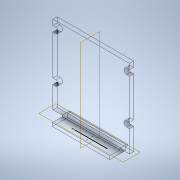
# Autodesk Inventor part: Xaar128
Saved by Autodesk Inventor 2022 (Build 260153000, 153)
## iProperties
Created: 2024-05-05
Part Number: Xaar128
Material: Generic
Document SubType Name: Modeling
Designer: raphael.hauk
Density: 1 g/cm^3
Appearance: Default
Author: raphael.hauk
Autodesk Inventor part; units mm, degrees
ref_plane "XY Plane" through (0, 0, 0) normal (0, 0, 1) x (1, 0, 0)
sketch "Sketch1" plane through (0, 0, 0) normal (0, 1, 0) x (-1, 0, 0)
  line L0 (0, -0.13) -> (17.417, -0.13)
  line L1 (17.417, -0.13) -> (17.417, 0.13)
  line L2 (17.417, 0.13) -> (0, 0.13)
  line L3 (0, 0.13) -> (0, -0.13)
  line L4 (-17.289, 0) -> (34.651, 0) construction
  line L5 (22.681, -3.5) -> (-5.169, -3.5)
  line L6 (-5.169, -3.5) -> (-5.169, 4)
  line L7 (-5.169, 4) -> (22.681, 4)
  line L8 (22.681, 4) -> (22.681, -3.5)
  line L9 (27.231, -2.85) -> (-9.869, -2.85) construction
  line L10 (-9.869, -2.85) -> (-9.869, -0.85) construction
  line L11 (-9.869, -0.85) -> (27.231, -0.85) construction
  line L12 (27.231, -0.85) -> (27.231, -2.85) construction
  point P0 (0, 0)
  dimension "d1" = 17.417
  dimension "d2" = 0.26
  dimension "d7" = 7.5
  dimension "d8" = 27.85
  dimension "d9" = 0.85
  dimension "d10" = 2
  dimension "d11" = 9.814
  dimension "d12" = 37.1
  dimension "d13" = 4.55
  dimension "d20" = 4.85
  constraints: 24 end point, 6 parallel, 3 horizontal, 3 perpendicular, 1 midpoint, 1 other
  measures "d1" distance of L0.start L0.end
  measures "d2" distance of L0.end L1.end
  measures "d7" distance of L7.end L5.start
  measures "d8" distance of L5.start L5.end
  measures "d9" distance between parallel lines of L11 L4
  measures "d10" distance of L9.end L10.end
  measures "d11" distance from line of L0.end L12
  measures "d12" distance of L9.start L9.end
  measures "d13" distance between parallel lines of L12 L8
  measures "d20" distance between parallel lines of L7 L11
ref_plane "Alu_Start_V" through (0, 2.27, 0) normal (0, 1, 0) x (-1, 0, 0)
sketch "Sketch2" plane through (0, 2.27, 0) normal (0, 1, 0) x (-1, 0, 0)
  line L0 (27.231, -2.85) -> (-9.869, -2.85) projected
  line L1 (27.231, -0.85) -> (27.231, -2.85) projected
  line L2 (-9.869, -0.85) -> (27.231, -0.85) projected
  line L3 (-9.869, -2.85) -> (-9.869, -0.85) projected
  point P0 (0, 0)
extrude "Extrusion2" add sketch "Sketch2" along normal blind 38
extrude "Extrusion3" add sketch "Sketch1" along normal blind 1.64 contours L3 L2 L1 L0 | L5 L6 L7 L8
sketch "Sketch3" plane through (0, 1.64, 0) normal (0, 1, 0) x (1, 0, 0)
  line L0 (5.169, 4.5) -> (-22.681, 4.5)
  line L1 (-22.681, 4.5) -> (-22.681, 0.85)
  line L2 (-22.681, 0.85) -> (5.169, 0.85)
  line L3 (5.169, 0.85) -> (5.169, 4.5)
  line L4 (9.869, 2.85) -> (-27.231, 2.85) construction
  line L5 (-27.231, 0.85) -> (9.869, 0.85) construction
  point P0 (0, 0)
  point P1 (-22.681, 3.5)
  point P2 (5.169, 3.5)
  point P3 (-22.681, 2.85)
  point P4 (5.169, 2.85)
  dimension "d22" = 3.65
  constraints: 8 end point, 3 point on line, 2 parallel, 1 horizontal, 1 perpendicular
  measures "d22" distance from line of L5 L0.start
extrude "Extrusion4" add sketch "Sketch3" along normal up to surface (0.63 mm away)
sketch "NozzleLine" plane through (0, 0, 0) normal (0, -1, 0) x (1, 0, 0)
  line L0 (0, 0) -> (-17.417, 0)
  point P0 (-17.417, 0.13)
  point P1 (-8.7085, 0)
  constraints: 2 end point, 1 horizontal, 1 midpoint, 1 vertical alignment
sketch "Sketch5" plane through (9.869, 40.27, -2.85) normal (0, 0, -1) x (-1, 0, 0)
  line L0 (0, -38) -> (0, 0) projected
  line L1 (0, -2.66) -> (1.35, -2.66)
  arc A0 (1.35, -5.36) -> (1.35, -2.66) centre (1.35, -4.01) ccw
  line L2 (1.35, -5.36) -> (0, -5.36)
  line L3 (37.1, 0) -> (0, 0) construction
  line L4 (4.7, -38) -> (32.55, -38) construction
  line L5 (37.1, -38) -> (37.1, 0) construction
  line L6 (18.55, 0) -> (18.55, -38) construction
  line L7 (37.1, -2.66) -> (35.75, -2.66)
  arc A1 (35.75, -2.66) -> (35.75, -5.36) centre (35.75, -4.01) ccw
  line L8 (35.75, -5.36) -> (37.1, -5.36)
  line L9 (0, -15.01) -> (36.8238, -15.01) construction
  line L10 (0, -27.36) -> (1.35, -27.36)
  arc A2 (1.35, -27.36) -> (1.35, -24.66) centre (1.35, -26.01) ccw
  line L11 (1.35, -24.66) -> (0, -24.66)
  line L12 (37.1, -30.02) -> (0, -30.02) construction
  line L13 (37.1, -27.36) -> (35.75, -27.36)
  arc A3 (35.75, -24.66) -> (35.75, -27.36) centre (35.75, -26.01) ccw
  line L14 (35.75, -24.66) -> (37.1, -24.66)
  line L15 (37.1, -2.66) -> (37.1, -5.36)
  line L16 (37.1, -24.66) -> (37.1, -27.36)
  point P0 (9.869, -40.27)
  point P1 (18.55, -30.02)
  dimension "d25" = 2.7
  dimension "d28" = 2.7
  dimension "d29" = 4.01
  dimension "d30" = 26.01
  constraints: 26 end point, 18 symmetric about line, 8 point on circle, 5 point on line, 4 centre point, 2 collinear, 2 horizontal, 2 midpoint, 2 perpendicular, 2 tangent, 3 other
  measures "d25" distance between parallel lines of L2 L1
  measures "d29" distance from line of L3 A1.centre
  measures "d30" distance from line of A3.centre L3
extrude "Extrusion5" cut sketch "Sketch5" against normal through all
ref_plane "NozzleLineCenter" through (-8.7085, 0, 0) normal (1, 0, 0) x (0, 1, 0)
body "Solid2"
